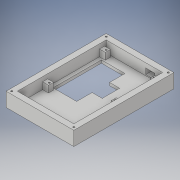
# Autodesk Inventor part: cabin_front
Saved by Autodesk Inventor 2019 (Build 230136000, 136)
## iProperties
Created: 2020-03-05
Part Number: cabin_front
Material: Generic
Document SubType Name: Modeling
Designer: laurenrhaylock
Density: 1 g/cm^3
Appearance: Default
Author: laurenrhaylock
Autodesk Inventor part; units mm, degrees
ref_plane "YZ Plane" through (0, 0, 0) normal (1, 0, 0) x (0, 1, 0)
ref_plane "XZ Plane" through (0, 0, 0) normal (0, 1, 0) x (-1, 0, 0)
ref_plane "XY Plane" through (0, 0, 0) normal (0, 0, 1) x (1, 0, 0)
sketch "Sketch1" plane through (0, 0, 0) normal (0, 1, 0) x (-1, 0, 0)
  line L0 (3.609, 163.5234) -> (-116.891, 163.5234)
  line L1 (-116.891, 163.5234) -> (-116.891, -14.4766)
  line L2 (-116.891, -14.4766) -> (3.609, -14.4766)
  line L3 (3.609, -14.4766) -> (3.609, 163.5234)
  dimension "d1" = 178
  dimension "d2" = 120.5
  constraints: 8 end point, 2 parallel, 1 horizontal, 1 perpendicular
  measures "d1" distance of L2.end L0.start
  measures "d2" distance of L0.start L0.end
extrude "Extrusion1" add sketch "Sketch1" along normal blind 25
sketch "Sketch2" plane through (0, 25, 0) normal (0, 1, 0) x (1, 0, 0)
  line L0 (6.391, -153.5234) -> (106.891, -153.5234)
  line L1 (106.891, -153.5234) -> (106.891, 4.4766)
  line L2 (106.891, 4.4766) -> (6.391, 4.4766)
  line L3 (6.391, 4.4766) -> (6.391, -153.5234)
  line L4 (-3.609, -163.5234) -> (116.891, -163.5234) projected
  line L5 (116.891, -163.5234) -> (116.891, 14.4766) projected
  point P0 (0, 0)
  dimension "d5" = 158
  dimension "d6" = 100.5
  dimension "d7" = 10
  dimension "d8" = 10
  constraints: 8 end point, 2 parallel, 1 horizontal, 1 perpendicular
  measures "d5" distance of L2.end L0.start
  measures "d6" distance of L0.start L0.end
  measures "d7" distance between parallel lines of L4 L0
  measures "d8" distance between parallel lines of L5 L1
extrude "Extrusion2" cut sketch "Sketch2" against normal blind 20
sketch "Sketch3" plane through (0, 5, 0) normal (0, 1, 0) x (1, 0, 0)
  line L0 (12.891, -96.5234) -> (54.891, -96.5234)
  line L1 (54.891, -96.5234) -> (54.891, -10.5234)
  line L2 (54.891, -10.5234) -> (12.891, -10.5234)
  line L3 (12.891, -10.5234) -> (12.891, -96.5234)
  line L4 (106.891, -153.5234) -> (6.391, -153.5234) projected
  line L5 (6.391, 4.4766) -> (106.891, 4.4766) projected
  line L6 (6.391, -153.5234) -> (6.391, 4.4766) projected
  line L7 (54.891, -69.0234) -> (72.891, -69.0234)
  line L8 (72.891, -69.0234) -> (72.891, -38.0234)
  line L9 (72.891, -38.0234) -> (54.891, -38.0234)
  line L10 (54.891, -38.0234) -> (54.891, -69.0234)
  line L11 (106.891, 4.4766) -> (106.891, -153.5234) projected
  line L12 (12.891, -55.0234) -> (106.891, -55.0234)
  point P0 (0, 0)
  dimension "d11" = 57
  dimension "d12" = 15
  dimension "d13" = 6.5
  dimension "d14" = 0
  dimension "d15" = 42
  dimension "d16" = 34
  dimension "d17" = 42.5
  dimension "d18" = 84.5
  dimension "d19" = 41.5
  dimension "d20" = 44.5
  dimension "d21" = 14
  constraints: 18 end point, 4 parallel, 3 horizontal, 2 perpendicular, 2 point on line
  measures "d11" distance between parallel lines of L4 L0
  measures "d12" distance between parallel lines of L5 L2
  measures "d13" distance between parallel lines of L6 L3
  measures "d14" distance between parallel lines of L1 L10
  measures "d15" distance between parallel lines of L3 L1
  measures "d16" distance between parallel lines of L11 L8
  measures "d17" distance between parallel lines of L5 L9
  measures "d18" distance between parallel lines of L4 L7
  measures "d19" distance between parallel lines of L0 L12
  measures "d20" distance between parallel lines of L2 L12
  measures "d21" distance between parallel lines of L7 L12
extrude "Extrusion3" cut sketch "Sketch3" against normal through all contours L3 L12 L1 L0 | L3 L2 L1 L12 | L1 L12 L8 L7 | L1 L9 L8 L12
sketch "Sketch4" plane through (0, 5, 0) normal (0, 1, 0) x (1, 0, 0)
  line L0 (6.391, -7.5234) -> (16.891, -7.5234)
  line L1 (16.891, -7.5234) -> (16.891, 1.4766)
  line L2 (16.891, 1.4766) -> (6.391, 1.4766)
  line L3 (6.391, 1.4766) -> (6.391, -7.5234)
  line L4 (6.391, -153.5234) -> (6.391, 4.4766) projected
  line L5 (6.391, 4.4766) -> (106.891, 4.4766) projected
  line L6 (6.391, -153.5234) -> (6.391, 4.4766) projected
  line L7 (6.391, -53.5234) -> (106.891, -53.5234)
  line L8 (12.891, -10.5234) -> (54.891, -10.5234) projected
  line L9 (6.391, -99.5234) -> (16.891, -99.5234)
  line L10 (16.891, -99.5234) -> (16.891, -108.5234)
  line L11 (16.891, -108.5234) -> (6.391, -108.5234)
  line L12 (6.391, -108.5234) -> (6.391, -99.5234)
  line L13 (106.891, -153.5234) -> (6.391, -153.5234) projected
  line L14 (56.641, -153.5234) -> (56.641, 4.4766)
  line L15 (6.391, 4.4766) -> (106.891, 4.4766) projected
  line L16 (-3.609, 14.4766) -> (-3.609, -163.5234) projected
  line L17 (106.891, -7.5234) -> (96.391, -7.5234)
  line L18 (96.391, -7.5234) -> (96.391, 1.4766)
  line L19 (96.391, 1.4766) -> (106.891, 1.4766)
  line L20 (106.891, 1.4766) -> (106.891, -7.5234)
  line L21 (108.391, -37.5234) -> (6.391, -37.5234)
  line L22 (106.891, -67.5234) -> (96.391, -67.5234)
  line L23 (106.891, -76.5234) -> (106.891, -67.5234)
  line L24 (96.391, -67.5234) -> (96.391, -76.5234)
  line L25 (96.391, -76.5234) -> (106.891, -76.5234)
  line L26 (54.891, -96.5234) -> (12.891, -96.5234) projected
  point P0 (0, 0)
  dimension "d24" = 0
  dimension "d25" = 10.5
  dimension "d26" = 9
  dimension "d27" = 3
  dimension "d28" = 43
  dimension "d29" = 60.25
  dimension "d30" = 30
  dimension "d37" = 43
  constraints: 36 end point, 12 symmetric about line, 4 perpendicular, 2 midpoint, 2 parallel, 2 point on line, 1 horizontal, 4 other
  measures "d24" distance between parallel lines of L4 L3
  measures "d25" distance of L1.end L2.end
  measures "d26" distance of L0.end L1.end
  measures "d27" distance between parallel lines of L5 L2
  measures "d28" distance between parallel lines of L8 L7
  measures "d29" distance between parallel lines of L16 L14
  measures "d30" distance between parallel lines of L17 L21
extrude "Extrusion4" add sketch "Sketch4" along normal blind 12 contours L3 L2 L1 L0 | L9 L10 L11 L4 | L17 L18 L19 L20 | L23 L25 L24 L22
sketch "Sketch6" plane through (0, 17, 0) normal (0, 1, 0) x (1, 0, 0)
  circle A0 centre (13.891, -3.0234) radius 1.5
  line L0 (6.391, -153.5234) -> (6.391, 4.4766) projected
  line L1 (16.891, 1.4766) -> (6.391, 1.4766) projected
  line L2 (6.391, -53.5234) -> (108.8142, -53.5234)
  line L3 (12.891, -10.5234) -> (54.891, -10.5234) projected
  line L4 (6.391, -108.5234) -> (16.891, -108.5234) projected
  circle A1 centre (13.891, -104.0234) radius 1.5
  line L5 (56.641, -153.5234) -> (56.641, 4.4766)
  line L6 (-3.609, 14.4766) -> (-3.609, -163.5234) projected
  circle A2 centre (99.391, -3.0234) radius 1.5
  line L7 (106.891, -7.5234) -> (106.891, -67.5234) projected
  line L8 (106.891, -37.5234) -> (6.391, -37.5234)
  line L9 (96.391, -7.5234) -> (106.891, -7.5234) projected
  circle A3 centre (99.391, -72.0234) radius 1.5
  line L10 (106.891, 4.4766) -> (106.891, -153.5234) projected
  line L11 (106.891, 1.4766) -> (96.391, 1.4766) projected
  point P0 (0, 0)
  dimension "d33" = 3
  dimension "d34" = 7.5
  dimension "d35" = 4.5
  dimension "d36" = 43
  dimension "d38" = 110
  dimension "d39" = 4.5
  dimension "d40" = 7.5
  dimension "d41" = 60.25
  dimension "d42" = 30
  dimension "d43" = 69
  dimension "d44" = 7.5
  dimension "d45" = 7.5
  dimension "d46" = 4.5
  constraints: 6 end point, 4 centre point, 3 symmetric about line, 2 point on line, 1 horizontal, 1 midpoint, 1 perpendicular, 1 vertical, 3 other
  measures "d33" diameter of A0
  measures "d34" distance from line of L0 A0.centre
  measures "d35" distance from line of L1 A0.centre
  measures "d36" distance between parallel lines of L3 L2
  measures "d38" distance between parallel lines of L1 L4
  measures "d39" distance from line of L4 A1.centre
  measures "d40" distance from line of L0 A1.centre
  measures "d41" distance between parallel lines of L6 L5
  measures "d42" distance between parallel lines of L9 L8
  measures "d43" distance of A2.centre A3.centre
  measures "d44" distance from line of L10 A3.centre
  measures "d45" distance from line of L10 A2.centre
  measures "d46" distance from line of L11 A2.centre
hole "Hole1" at (13.891, 17, 3.0234) at (13.891, 17, 104.0234) at (99.391, 17, 72.0234) at (99.391, 17, 3.0234) direction (0, -1, 0) diameter 3 depth 10 tip angle 118
thread "Thread1" size "M3x0.5" class "6H" standard "ANSI Metric M Profile" full length
thread "Thread2" size "M3x0.5" class "6H" standard "ANSI Metric M Profile" full length
thread "Thread3" size "M3x0.5" class "6H" standard "ANSI Metric M Profile" full length
thread "Thread4" size "M3x0.5" class "6H" standard "ANSI Metric M Profile" full length
sketch "Sketch7" plane through (0, 25, 0) normal (0, 1, 0) x (1, 0, 0)
  circle A0 centre (1.391, -158.5234) radius 1.5
  line L0 (-3.609, -163.5234) -> (116.891, -163.5234) projected
  line L1 (-3.609, 14.4766) -> (-3.609, -163.5234) projected
  line L2 (-3.609, 14.4766) -> (-3.609, -163.5234) projected
  line L3 (-3.609, -74.5234) -> (116.891, -74.5234)
  line L4 (116.891, -163.5234) -> (116.891, 14.4766) projected
  circle A1 centre (1.391, 9.4766) radius 1.5
  line L5 (56.641, -163.5234) -> (56.641, 14.4766)
  line L6 (116.891, 14.4766) -> (-3.609, 14.4766) projected
  circle A2 centre (111.891, -158.5234) radius 1.5
  circle A3 centre (111.891, 9.4766) radius 1.5
  point P0 (0, 0)
  dimension "d62" = 3
  dimension "d63" = 5
  dimension "d64" = 5
  dimension "d65" = 89
  dimension "d66" = 60.25
  constraints: 4 centre point, 4 end point, 4 midpoint, 3 symmetric about line, 1 horizontal, 1 vertical, 3 other
  measures "d62" diameter of A0
  measures "d63" distance from line of L0 A0.centre
  measures "d64" distance from line of L1 A0.centre
  measures "d65" distance between parallel lines of L0 L3
  measures "d66" distance between parallel lines of L1 L5
hole "Hole2" at (1.391, 25, 158.5234) at (1.391, 25, -9.4766) at (111.891, 25, -9.4766) at (111.891, 25, 158.5234) direction (0, -1, 0) diameter 3 depth 20 tip angle 118
thread "Thread5" size "M3x0.5" class "6H" standard "ANSI Metric M Profile" full length
thread "Thread6" size "M3x0.5" class "6H" standard "ANSI Metric M Profile" full length
thread "Thread7" size "M3x0.5" class "6H" standard "ANSI Metric M Profile" full length
thread "Thread8" size "M3x0.5" class "6H" standard "ANSI Metric M Profile" full length
sketch "Sketch8" plane through (6.391, 25, -4.4766) normal (0, 0, 1) x (1, 0, 0)
  line L0 (70.5, -18) -> (86.5, -18)
  line L1 (86.5, -18) -> (86.5, -8)
  line L2 (86.5, -8) -> (70.5, -8)
  line L3 (70.5, -8) -> (70.5, -18)
  line L4 (100.5, 0) -> (100.5, -20) projected
  line L5 (0, 0) -> (100.5, 0) projected
  line L6 (0, -20) -> (100.5, -20) projected
  point P0 (-6.391, -25)
  dimension "d82" = 14
  dimension "d83" = 16
  dimension "d84" = 8
  dimension "d85" = 2
  constraints: 8 end point, 2 parallel, 1 horizontal, 1 perpendicular
  measures "d82" distance between parallel lines of L4 L1
  measures "d83" distance between parallel lines of L3 L1
  measures "d84" distance between parallel lines of L5 L2
  measures "d85" distance between parallel lines of L6 L0
extrude "Extrusion5" cut sketch "Sketch8" against normal through all
body "Solid1"
